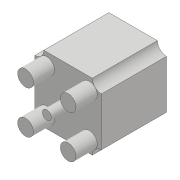
# Autodesk Inventor part: VRUZEND_Caps
Saved by Autodesk Inventor 2018 (Build 220112000, 112)
## iProperties
Created: 2019-09-04
Part Number: VRUZEND_Caps
Material: Generic
Document SubType Name: Modeling
Designer: Clevo
Density: 1 g/cm^3
Appearance: Default
Author: Clevo
Autodesk Inventor part; units mm, degrees
ref_plane "YZ Plane" through (0, 0, 0) normal (1, 0, 0) x (0, 1, 0)
ref_plane "XZ Plane" through (0, 0, 0) normal (0, 1, 0) x (-1, 0, 0)
ref_plane "XY Plane" through (0, 0, 0) normal (0, 0, 1) x (1, 0, 0)
sketch "Sketch1" plane through (0, 0, 0) normal (0, 1, 0) x (-1, 0, 0)
  line L0 (-11, 11) -> (11, 11)
  line L1 (11, 11) -> (11, -11)
  line L2 (11, -11) -> (-11, -11)
  line L3 (-11, -11) -> (-11, 11)
  line L4 (-11, 11) -> (11, -11) construction
  line L5 (11, 11) -> (-11, -11) construction
  point P0 (0, 0)
  dimension "d0" = 22
  dimension "d1" = 22
  constraints: 12 end point, 2 midpoint, 2 parallel, 1 horizontal, 1 perpendicular
  measures "d0" distance of L0.end L1.end
  measures "d1" distance of L0.start L0.end
extrude "Extrusion1" add sketch "Sketch1" along normal blind 28.5
sketch "Sketch2" plane through (0, 28.5, 0) normal (0, 1, 0) x (1, 0, 0)
  circle A0 centre (0, 0) radius 9
  dimension "d4" = 18
  constraints: 1 centre point, 1 coincident
  measures "d4" diameter of A0
extrude "Extrusion2" cut sketch "Sketch2" against normal blind 14.5
sketch "Sketch3" plane through (0, 0, 0) normal (0, -1, 0) x (1, 0, 0)
  line L0 (11, 11) -> (-11, 11) projected
  line L1 (-11, 11) -> (-11, -11) projected
  line L2 (-11, -11) -> (11, -11) projected
  line L3 (11, -11) -> (11, 11) projected
  line L4 (11, 11) -> (11, -11) projected
  circle A0 centre (11, -11) radius 3
  line L5 (11, -11) -> (-11, -11) projected
  circle A1 centre (-11, -11) radius 3
  line L6 (-11, 11) -> (11, 11) projected
  circle A2 centre (-11, 11) radius 3
  circle A3 centre (11, 11) radius 3
  point P0 (0, 0)
  dimension "d7" = 6
  dimension "d8" = 6
  dimension "d9" = 6
  dimension "d10" = 6
  constraints: 4 centre point, 4 coincident
  measures "d7" diameter of A0
  measures "d8" diameter of A1
  measures "d9" diameter of A2
  measures "d10" diameter of A3
extrude "Extrusion3" cut sketch "Sketch3" against normal through all contours A2 L1 L0 | L0 L1 A2 | A3 L3 L0 | L0 L3 A3 | A1 L2 L1 | L1 L2 A1 | A0 L2 L3 | L3 L2 A0
sketch "Sketch4" plane through (0, 0, 0) normal (0, -1, 0) x (1, 0, 0)
  circle A0 centre (0, 0) radius 1.5
  arc A1 (8, 11) -> (11, 8) centre (11, 11) ccw projected
  line L0 (8, 11) -> (-8, 11) projected
  arc A2 (-11, 8) -> (-8, 11) centre (-11, 11) ccw projected
  line L1 (-11, 8) -> (-11, -8) projected
  arc A3 (-8, -11) -> (-11, -8) centre (-11, -11) ccw projected
  line L2 (-8, -11) -> (8, -11) projected
  arc A4 (11, -8) -> (8, -11) centre (11, -11) ccw projected
  line L3 (11, -8) -> (11, 8) projected
  line L4 (7.0402, 7.0402) -> (4.4402, 7.0402)
  line L5 (-7.0402, 7.0402) -> (-7.0402, 4.4402)
  line L6 (-7.0402, -7.0402) -> (-4.4402, -7.0402)
  line L7 (7.0402, -7.0402) -> (7.0402, -4.4402)
  line L8 (7.0402, 7.0402) -> (-7.0402, -7.0402) construction
  line L9 (-7.0402, 7.0402) -> (7.0402, -7.0402) construction
  circle A5 centre (-7.0402, -7.0402) radius 2.6
  circle A6 centre (-7.0402, 7.0402) radius 2.6
  circle A7 centre (7.0402, 7.0402) radius 2.6
  circle A8 centre (7.0402, -7.0402) radius 2.6
  line L10 (-4.4402, -7.0402) -> (4.4402, -7.0402)
  line L11 (-7.0402, 4.4402) -> (-7.0402, -4.4402)
  line L12 (-7.0402, -4.4402) -> (-7.0402, -7.0402)
  line L13 (4.4402, -7.0402) -> (7.0402, -7.0402)
  line L14 (7.0402, -4.4402) -> (7.0402, 4.4402)
  line L15 (7.0402, 4.4402) -> (7.0402, 7.0402)
  line L16 (4.4402, 7.0402) -> (-4.4402, 7.0402)
  line L17 (-4.4402, 7.0402) -> (-7.0402, 7.0402)
  dimension "d13" = 3
  dimension "d15" = 14.0804
  dimension "d16" = 5.2
  dimension "d17" = 5.2
  dimension "d18" = 5.2
  dimension "d19" = 5.2
  dimension "d20" = 14.0804
  constraints: 28 end point, 18 parallel, 9 perpendicular, 8 point on circle, 5 centre point, 5 coincident, 3 horizontal, 2 midpoint, 1 tangent
  measures "d13" diameter of A0
  measures "d15" distance of L5.start L6.start
  measures "d16" diameter of A5
  measures "d17" diameter of A6
  measures "d18" diameter of A7
  measures "d19" diameter of A8
  measures "d20" distance of L6.start L7.start
extrude "Extrusion4" cut sketch "Sketch4" against normal blind 7 contours A1 A7 L16 A6 A2 L0 | A1 L3 A4 A8 L14 A7 | A7 L14 A8 L10 A5 L11 A6 L16 | A6 L11 A5 A3 L1 A2 | A4 L2 A3 A5 L10 A8
equation "\"d1\" = d0"
equation "\"d15\" = d20"
equation "\"d17\" = d16"
equation "\"d18\" = d17"
equation "\"d19\" = d18"
body "Solid1"
